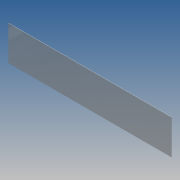
# Autodesk Inventor part: screen
Saved by Autodesk Inventor 2013 SP2 (Build 170200200, 200)
## iProperties
Company: HERA Project
Created: 2013-05-31
Part Number: screen
Material: Glass
Document SubType Name: Modeling
Designer: David DeBoer
Density: 2.18 g/cm^3
Description: Screen
Mass: 332232 g
Surface Area: 1.20097e+06 cm^2
Volume: 152400 cm^3
Author: David DeBoer
Title: Screen
Autodesk Inventor part; units mm, degrees
ref_plane "YZ Plane" through (0, 0, 0) normal (1, 0, 0) x (0, 1, 0)
ref_plane "XZ Plane" through (0, 0, 0) normal (0, 1, 0) x (-1, 0, 0)
ref_plane "XY Plane" through (0, 0, 0) normal (0, 0, 1) x (1, 0, 0)
sketch "Sketch2" plane through (0, 0, 0) normal (0, 0, 1) x (1, 0, 0)
  line L0 (0, 0) -> (10160, 0)
  line L1 (10160, 0) -> (10160, 2159)
  line L2 (10160, 2159) -> (0, 2159)
  line L3 (0, 2159) -> (0, 0)
  dimension "d4" = 10160
  dimension "d5" = 2159
  constraints: 8 end point, 2 parallel, 1 horizontal, 1 perpendicular
  measures "d4" distance of L0.start L0.end
  measures "d5" distance of L2.end L0.start
extrude "Extrusion2" add sketch "Sketch2" along normal blind 25.4
body "Solid2"
